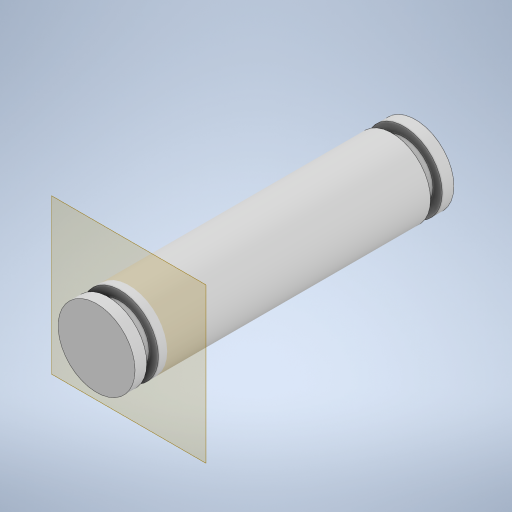
# Autodesk Inventor part: axle-upper
Saved by Autodesk Inventor 2024 (Build 280153000, 153)
## iProperties
Created: 2024-04-13
Part Number: axle-upper
Material: Generic
Document SubType Name: Modeling
Designer: MaartenGeorgesBuelen
Density: 1 g/cm^3
Appearance: Default
Author: MaartenGeorgesBuelen
## iProperties of the stored document axle-upper_3DPrint.ipt
Created: 2024-04-13
Part Number: axle-upper_3DPrint
Material: Generic
Document SubType Name: Modeling
Designer: MaartenGeorgesBuelen
Density: 1 g/cm^3
Appearance: Default
Author: MaartenGeorgesBuelen
Autodesk Inventor part; units mm, degrees
ref_plane "YZ Plane" through (0, 0, 0) normal (1, 0, 0) x (0, 1, 0)
ref_plane "Work Plane1" through (0, 0, 0) normal (0, 0, 1) x (1, 0, 0)
sketch "Sketch1" plane through (0, 0, 0) normal (0, 0, 1) x (1, 0, 0)
  circle A0 centre (0, -19) radius 4.7
  circle A1 centre (19, 0) radius 4.7
  circle A2 centre (0, 19) radius 4.7
  circle A3 centre (-19, 0) radius 4.7
  circle A4 centre (0, 0) radius 13.5
  circle A5 centre (-13.435, 13.435) radius 4.7
  circle A6 centre (13.435, 13.435) radius 4.7
  circle A7 centre (13.435, -13.435) radius 4.7
  circle A8 centre (-13.435, -13.435) radius 4.7
  circle A9 centre (0, 0) radius 13.15
  point P0 (0, 0)
  dimension "d0" = 0.35
  dimension "d16" = 9.4
  dimension "d17" = 27
  dimension "d18" = 14.542
  dimension "d19" = 14.542
  dimension "d20" = 26.8701
  dimension "d21" = 19
  dimension "d22" = 26.8701
  dimension "d23" = 35.1074
  dimension "d24" = 38
  dimension "d25" = 26.8701
  dimension "d26" = 14.542
  dimension "d27" = 19
  dimension "d28" = 35.1074
  dimension "d29" = 26.8701
  dimension "d30" = 35.1074
  dimension "d31" = 38
  dimension "d32" = 26.8701
  constraints: 10 centre point, 7 equal radius
  measures "d0" radial gap between concentric circles of A4 A9
  measures "d16" diameter of A1
  measures "d17" diameter of A4
  measures "d18" distance of A1.centre A6.centre
  measures "d19" distance of A1.centre A7.centre
  measures "d20" distance of A1.centre A2.centre
  measures "d21" distance of A1.centre A4.centre
  measures "d22" distance of A1.centre A0.centre
  measures "d23" distance of A1.centre A8.centre
  measures "d24" distance of A1.centre A3.centre
  measures "d25" distance of A6.centre A7.centre
  measures "d26" distance of A6.centre A2.centre
  measures "d27" distance of A6.centre A4.centre
  measures "d28" distance of A6.centre A0.centre
  measures "d29" distance of A6.centre A5.centre
  measures "d30" distance of A6.centre A3.centre
  measures "d31" distance of A7.centre A5.centre
  measures "d32" distance of A7.centre A8.centre
ref_plane "Work Plane2" through (-20, -20, -70) normal (0, 0, -1) x (0, 1, 0)
ref_plane "Work Plane3" through (-25, -81.8654, -89) normal (0, 0, -1) x (0, 1, 0)
extrude "Extrusion1" add sketch "Sketch1" against normal blind 90 contours A9
move faces "Move1" translate (0, 0, 3) faces at (-4.0086, 0.988, 0)
sketch "Sketch5" plane through (0, 0, 3) normal (0, 0, 1) x (1, 0, 0)
  circle A0 centre (0, 0) radius 10
  point P0 (0, 0)
  dimension "d11" = 20
  constraints: 1 centre point, 1 coincident
  measures "d11" diameter of A0
extrude "Extrusion4" add sketch "Sketch5" along normal blind 4
sketch "Sketch6" plane through (0, 0, 7) normal (0, 0, 1) x (1, 0, 0)
  circle A0 centre (0, 0) radius 13.15 projected
  point P0 (0, 0)
extrude "Extrusion5" add sketch "Sketch6" along normal blind 4
sketch "Sketch7" plane through (0, 0, -90) normal (0, 0, -1) x (-1, 0, 0)
  circle A0 centre (0, 0) radius 13.15 projected
  circle A1 centre (0, 0) radius 10
  point P0 (0, 0)
  dimension "d35" = 20
  constraints: 1 centre point
  measures "d35" diameter of A1
extrude "Extrusion6" add sketch "Sketch7" along normal blind 4 contours A1
sketch "Sketch8" plane through (0, 0, -94) normal (0, 0, -1) x (-1, 0, 0)
  circle A0 centre (0, 0) radius 13.15 projected
  point P0 (0, 0)
extrude "Extrusion7" add sketch "Sketch8" along normal blind 4
body "Solid1"
